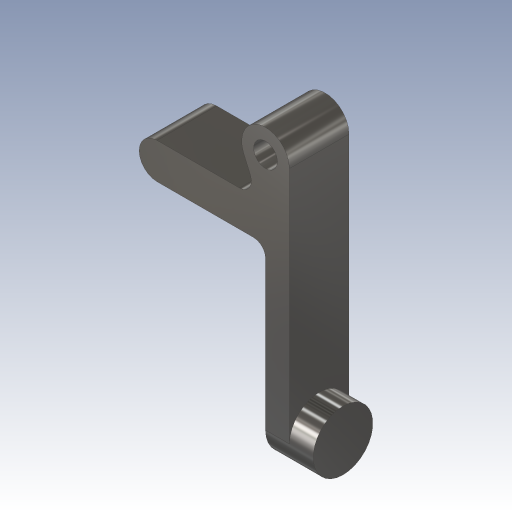
# Autodesk Inventor part: BT017_huenin20_23
Saved by Autodesk Inventor 2023.3 (Build 273359000, 359)
## iProperties
Company: HTBLA Kaindorf
RuleStatus: InUse
Created: 2024-01-29
Part Number: BT017_huenin20_23
Project: Fiberprinter-Hotend
Material: Stahl
Description: SMN_Aktuatorhebel
Document SubType Name: Modeling
Designer: huenin20
Density: 7.85 g/cm^3
Appearance: Stahl - poliert
Mass: 3.58833 g
Surface Area: 5.78997 cm^2
Volume: 0.457112 cm^3
AfterDocNew0: iProperties-Editor_aufrufen
Author: nicob
Keywords: 2023
Autodesk Inventor part; units mm, degrees
ref_plane "YZ Plane" through (0, 0, 0) normal (1, 0, 0) x (0, 1, 0)
ref_plane "XZ Plane" through (0, 0, 0) normal (0, 1, 0) x (-1, 0, 0)
ref_plane "XY Plane" through (0, 0, 0) normal (0, 0, 1) x (1, 0, 0)
sketch "Skizze3" plane through (0, 0, 0) normal (1, 0, 0) x (0, 1, 0)
  circle A0 centre (0, 0) radius 1
  circle A1 centre (0, 0) radius 2
  line L0 (2, 0) -> (2, -5)
  line L1 (0, -22.5) -> (0, -5)
  line L2 (0, -5) -> (-1.833, -0.8)
  line L3 (2, -5) -> (2, -17.5)
  line L4 (2, -17.5) -> (4, -17.5)
  line L5 (4, -17.5) -> (4, -22.5)
  line L6 (4, -22.5) -> (0, -22.5)
  line L7 (-0.6547, -3.5) -> (-9.1, -3.5)
  line L8 (-10.6, -5) -> (-10.6, -5)
  line L9 (-9.1, -6.5) -> (0, -6.5)
  arc A2 (-9.1, -3.5) -> (-10.6, -5) centre (-9.1, -5) ccw
  arc A3 (-10.6, -5) -> (-9.1, -6.5) centre (-9.1, -5) ccw
  point P0 (4, -20)
  point P1 (-10.6, -5)
  point P2 (-10.6, -5)
  dimension "d4" = 2
  dimension "d5" = 4
  dimension "d8" = 5
  dimension "d9" = 2
  dimension "d10" = 5
  dimension "d11" = 20
  dimension "d12" = 2
  dimension "d16" = 5
  dimension "d17" = 3
  dimension "d18" = 10.6
  dimension "d19" = 1.5
  constraints: 20 end point, 6 point on circle, 6 tangent, 5 perpendicular, 4 centre point, 2 coincident, 2 midpoint, 2 point on line, 1 concentric, 1 horizontal, 1 horizontal alignment, 1 vertical, 1 vertical alignment
  measures "d4" diameter of A0
  measures "d5" diameter of A1
  measures "d8" distance of point (0, 0) L1.end
  measures "d9" distance between parallel lines of L1 L3
  measures "d10" distance between parallel lines of L6 L4
  measures "d11" vertical distance of point (0, 0) point (4, -20)
  measures "d12" distance between parallel lines of L3 L5
  measures "d16" vertical distance of point (0, 0) point (-10.6, -5)
  measures "d17" distance between parallel lines of L9 L7
  measures "d18" distance between parallel lines of L1 L8
  measures "d19" radius of A2
extrude "Extrusion3" add sketch "Skizze3" along normal blind 5
fillet "Rundung1" radius 2.5 4 edges at (0, 3, -17.5) (5, 3, -17.5) (5, 2, -22.5) (0, 2, -22.5)
fillet "Rundung2" radius 1 2 edges at (2.5, -0.6547, -3.5) (2.5, 0, -6.5)
